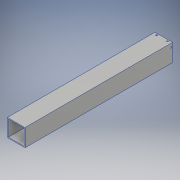
# Autodesk Inventor part: TelescopeNewOuter
Saved by Autodesk Inventor 2018.3 (Build 223284000, 284)
## iProperties
Created: 2020-01-19
Part Number: TelescopeNewOuter
Material: Aluminum 6061
Document SubType Name: Modeling
Designer: Cooper
Density: 2.7 g/cm^3
Appearance: Aluminum - Flat
Mass: 1091.51 g
Surface Area: 2566.01 cm^2
Volume: 404.263 cm^3
Author: Cooper
Autodesk Inventor part; units mm, degrees
ref_plane "YZ Plane" through (0, 0, 0) normal (1, 0, 0) x (0, 1, 0)
ref_plane "XZ Plane" through (0, 0, 0) normal (0, 1, 0) x (-1, 0, 0)
ref_plane "XY Plane" through (0, 0, 0) normal (0, 0, 1) x (1, 0, 0)
sketch "Sketch1" plane through (0, 0, 0) normal (0, 0, 1) x (1, 0, 0)
  line L0 (0, 0) -> (63.5, 0)
  line L1 (63.5, 0) -> (63.5, 63.5)
  line L2 (63.5, 63.5) -> (0, 63.5)
  line L3 (0, 63.5) -> (0, 0)
  line L4 (3.175, 60.325) -> (60.325, 60.325)
  line L5 (60.325, 60.325) -> (60.325, 3.175)
  line L6 (60.325, 3.175) -> (3.175, 3.175)
  line L7 (3.175, 3.175) -> (3.175, 60.325)
  dimension "d0" = 63.5
  dimension "d1" = 63.5
  dimension "d2" = 3.175
  constraints: 16 end point, 4 parallel, 2 perpendicular, 1 horizontal, 3 other
  measures "d0" distance of L2.end L0.start
  measures "d1" distance of L0.start L0.end
  measures "d2" distance between parallel lines of L2 L4
extrude "Extrusion1" add sketch "Sketch1" along normal blind 533.4
sketch "Sketch3" plane through (0, 63.5, 0) normal (0, 1, 0) x (1, 0, 0)
  line L0 (9.525, 0) -> (9.525, -25.4)
  line L1 (9.525, -25.4) -> (53.975, -25.4)
  line L2 (53.975, -25.4) -> (53.975, 0)
  line L3 (63.5, 0) -> (63.5, -533.4) projected
  line L4 (63.5, 0) -> (0, 0) projected
  line L5 (9.525, 0) -> (53.975, 0)
  line L6 (0, 0) -> (63.5, 0) projected
  line L7 (63.5, 0) -> (0, 0) projected
  line L8 (0, 0) -> (0, -533.4) projected
  line L9 (63.5, -533.4) -> (0, -533.4) projected
  line L10 (63.5, 0) -> (63.5, -533.4) projected
  dimension "d14" = 44.45
  dimension "d16" = 25.4
  dimension "d19" = 9.525
  dimension "d20" = 9.525
  constraints: 8 end point, 3 perpendicular, 2 parallel, 1 collinear, 1 point on line, 1 vertical
  measures "d14" distance of L0.end L1.end
  measures "d16" distance of L1.end L2.end
  measures "d19" distance between parallel lines of L3 L2
  measures "d20" distance between parallel lines of L8 L0
extrude "Extrusion2" cut sketch "Sketch3" against normal blind 63.5 contours L4 L2 L1 L0
sketch "Sketch5" plane through (0, 63.5, 533.4) normal (0, 1, 0) x (1, 0, 0)
  line L0 (53.975, 508) -> (9.525, 508) projected
  line L1 (53.975, 533.4) -> (53.975, 508) projected
  line L2 (9.525, 508) -> (9.525, 533.4) projected
  line L3 (53.975, 533.4) -> (9.525, 533.4)
  point P0 (0, 533.4)
  constraints: 2 end point, 1 perpendicular
extrude "Extrusion3" add sketch "Sketch5" against normal blind 3.175
sketch "Sketch6" plane through (0, 63.5, 0) normal (0, 1, 0) x (1, 0, 0)
  line L0 (0, 0) -> (0, -533.4) projected
  line L1 (63.5, 0) -> (63.5, -533.4) projected
  line L2 (63.5, 0) -> (0, 0) projected
  point P0 (12.192, -6.35)
  point P1 (51.308, -6.35)
  dimension "d23" = 12.192
  dimension "d24" = 12.192
  dimension "d25" = 6.35
  constraints: 1 horizontal alignment
  measures "d23" distance from line of L0 point (12.192, -6.35)
  measures "d24" distance from line of L1 point (51.308, -6.35)
  measures "d25" distance from line of L2 point (51.308, -6.35)
hole "Hole2" at (12.192, 63.5, 6.35) at (51.308, 63.5, 6.35) direction (0, -1, 0) diameter 5.1562 depth 25.4 tip angle 118
sketch "Sketch7" plane through (63.5, 0, 0) normal (1, 0, 0) x (0, 0, -1)
  line L0 (0, 63.5) -> (-533.4, 63.5) projected
  line L1 (0, 0) -> (0, 63.5) projected
  point P0 (-6.35, 51.308)
  dimension "d33" = 12.192
  dimension "d34" = 6.35
  measures "d33" distance from line of L0 point (-6.35, 51.308)
  measures "d34" distance from line of L1 point (-6.35, 51.308)
hole "Hole3" at (63.5, 51.308, 6.35) direction (-1, 0, 0) diameter 5.1562 depth 76.2 tip angle 118
equation "\"d19\" = d20"
equation "\"d24\" = d23"
body "Solid1"
